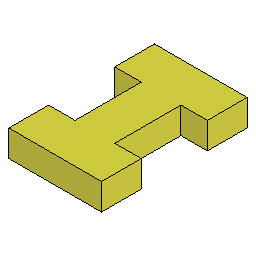
Prindere Masa (Autodesk Fusion 360 design; units mm, degrees)
part number: 2026-06-02-22-23-08-209
Autodesk Fusion 360 part; units mm, degrees
sketch "Sketch1" plane through (0, 0, 0) normal (0, 0, 1) x (1, 0, 0)
  line L0 (230, 0) -> (230, -6)
  line L1 (230, -6) -> (234, -6)
  line L2 (234, -6) -> (234, -10)
  line L3 (234, -10) -> (222, -10)
  line L4 (222, -10) -> (222, -6)
  line L5 (222, -6) -> (226, -6)
  line L6 (226, -6) -> (226, 0)
  line L7 (226, 0) -> (230, 0)
  line L8 (230, 6) -> (234, 6)
  line L9 (234, 6) -> (234, 10)
  line L10 (234, 10) -> (222, 10)
  line L11 (222, 10) -> (222, 6)
  line L12 (222, 6) -> (226, 6)
  line L13 (226, 6) -> (226, 0)
  line L14 (230, 0) -> (230, 6)
  line L15 (229, 0) -> (229, 7)
  line L16 (229, 7) -> (233, 7)
  line L17 (233, 7) -> (233, 9)
  line L18 (233, 9) -> (223, 9)
  line L19 (223, 9) -> (223, 7)
  line L20 (223, 7) -> (227, 7)
  line L21 (227, 7) -> (227, 0)
  line L22 (229, 0) -> (229, -7)
  line L23 (229, -7) -> (233, -7)
  line L24 (233, -7) -> (233, -9)
  line L25 (233, -9) -> (223, -9)
  line L26 (223, -9) -> (223, -7)
  line L27 (223, -7) -> (227, -7)
  line L28 (227, -7) -> (227, 0)
  line L29 (235, -5) -> (235, -11)
  line L30 (235, -11) -> (221, -11)
  line L31 (221, -11) -> (221, -5)
  line L32 (221, -5) -> (225, -5)
  line L33 (225, -5) -> (225, 0)
  line L34 (225, 5) -> (225, 0)
  line L35 (221, 5) -> (225, 5)
  line L36 (221, 11) -> (221, 5)
  line L37 (235, 11) -> (221, 11)
  line L38 (235, 5) -> (235, 11)
  line L39 (231, 5) -> (235, 5)
  line L40 (231, 0) -> (231, 5)
  line L41 (231, 0) -> (231, -5)
  line L42 (231, -5) -> (235, -5)
  dimension "d775" = 6
  dimension "d776" = 4
  dimension "d777" = 12
  dimension "d778" = 4
  dimension "d779" = 4
  dimension "d780" = 4
  dimension "d781" = -1
  dimension "d782" = 1
  dimension "d783" = 1
  constraint vertical L0
  constraint perpendicular L0 L1
  constraint perpendicular L1 L2
  constraint perpendicular L2 L3
  constraint perpendicular L3 L4
  constraint perpendicular L4 L5
  constraint perpendicular L5 L6
  constraint perpendicular L0 L7
  constraint symmetric L0.start L7 L14.start
  constraint symmetric L0.end L7 L8.start
  constraint symmetric L1.end L7 L8.end
  constraint symmetric L2.end L7 L9.end
  constraint symmetric L3.end L7 L10.end
  constraint symmetric L4.end L7 L11.end
  constraint symmetric L5.end L7 L12.end
  constraint symmetric L6.end L7 L13.end
  constraint coincident L21.end L28.end
  constraint coincident L15.start L22.start
  constraint coincident L7 L15.start
  constraint coincident L7 L21.end
  constraint horizontal L6.end L33.end
  constraint horizontal L0.start L40.start
  measures "d775" distance of L0.start L0.end
  measures "d776" distance of L0.end L1.end
  measures "d777" distance of L2.end L3.end
  measures "d778" distance of L1.end L2.end
  measures "d779" distance of L3.end L4.end
  measures "d780" distance of L0.start L6.end
extrude "Extrude1" add sketch "Sketch1" along normal blind 4 contours L7 L22 L23 L24 L25 L26 L27 L28 | L7 L15 L16 L17 L18 L19 L20 L21 | L29 L30 L31 L32 L33 L34 L35 L36 L37 L38 L39 L40 L41 L42 makes body 1 at (226, -10.6667, 0) makes body 2 at (227.6667, -8.3333, 0)
extrude "Extrude2" add sketch "Sketch1" along normal blind 2 from surface at 2 contours L0 L1 L2 L3 L4 L5 L6 L7 L22 L23 L24 L25 L26 L27 L28 | L7 L8 L9 L10 L11 L12 L13 L14 L15 L16 L17 L18 L19 L20 L21 bodies 1 2
named bodies: "Poarta Dreapta Sus"
